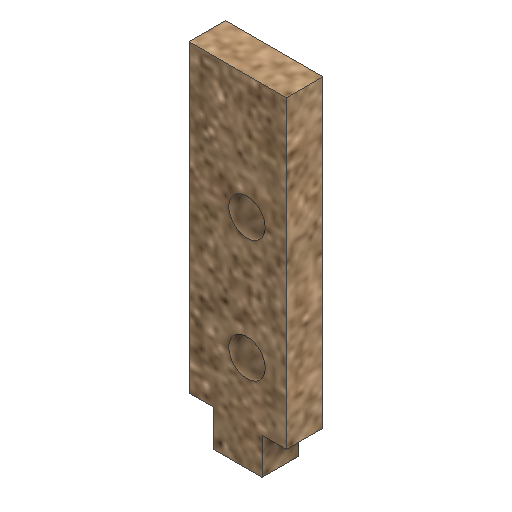
# Autodesk Inventor part: test_side2
Saved by Autodesk Inventor 2024 (Build 280153000, 153)
## iProperties
Created: 2024-05-27
Part Number: test_side2
Material: MDF Medium Density Fiberboard
Document SubType Name: Modeling
Designer: op04o
Density: 0.8 g/cm^3
Appearance: Cardboard - Corrugated
Mass: 0.474871 g
Surface Area: 6.68274 cm^2
Volume: 0.593588 cm^3
Author: op04o
Autodesk Inventor part; units mm, degrees
ref_plane "YZ Plane" through (0, 0, 0) normal (1, 0, 0) x (0, 1, 0)
ref_plane "XZ Plane" through (0, 0, 0) normal (0, 1, 0) x (-1, 0, 0)
ref_plane "XY Plane" through (0, 0, 0) normal (0, 0, 1) x (1, 0, 0)
sketch "Sketch1" plane through (0, 0, 0) normal (0, 0, 1) x (1, 0, 0)
  line L0 (-4, -12.5) -> (4, -12.5)
  line L1 (4, -12.5) -> (4, 12.5)
  line L2 (4, 12.5) -> (-4, 12.5)
  line L3 (-4, 12.5) -> (-4, -12.5)
  line L4 (-4, -12.5) -> (4, 12.5) construction
  line L5 (4, -12.5) -> (-4, 12.5) construction
  line L6 (-2, -12.5) -> (2, -12.5)
  line L7 (2, -12.5) -> (2, -15.5)
  line L8 (2, -15.5) -> (-2, -15.5)
  line L9 (-2, -15.5) -> (-2, -12.5)
  circle A0 centre (0.768, 2.4) radius 1.5
  circle A1 centre (0.768, -7.6) radius 1.5
  point P0 (0, 0)
  point P1 (0, -15.5)
  point P2 (0, -12.5)
  point P3 (0, 12.5)
  dimension "d0" = 25
  dimension "d1" = 8
  dimension "d2" = 3
  dimension "d3" = 4
  dimension "d9" = 3
  dimension "d10" = 10.1
  dimension "d11" = 3
  dimension "d12" = 10
  constraints: 20 end point, 5 midpoint, 4 parallel, 2 centre point, 2 horizontal, 2 perpendicular, 2 point on line, 2 vertical alignment
  measures "d0" distance of L0.end L1.end
  measures "d1" distance of L1.end L2.end
  measures "d2" distance of L6.end L7.end
  measures "d3" distance of L7.end L8.end
  measures "d9" diameter of A0
  measures "d10" distance from line of A0.centre L2
  measures "d11" diameter of A1
  measures "d12" distance of A1.centre A0.centre
extrude "Extrusion1" add sketch "Sketch1" along normal blind 3
body "Solid1"
